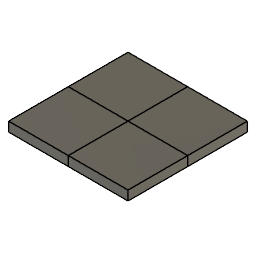
Tile_Base_V1 (Autodesk Fusion 360 design; units mm, degrees)
part number: 2026-04-30-04-34-27-327
Autodesk Fusion 360 part; units mm, degrees
note: some values were not read from the file. Chosen so that the rebuilt part matches the saved one: which bodies a step acts on.
sketch "Sketch1" plane through (0, 0, 0) normal (0, 0, 1) x (1, 0, 0)
  line L0 (-25, 25) -> (25, 25)
  line L1 (25, 25) -> (25, -25)
  line L2 (25, -25) -> (-25, -25)
  line L3 (-25, -25) -> (-25, 25)
  constraint horizontal L0
  constraint vertical L1
  constraint horizontal L2
  constraint vertical L3
extrude "Extrude1" add sketch "Sketch1" along normal blind 5 makes body 1
sketch "Sketch2" plane through (0, -25, 0) normal (0, -1, 0) x (1, 0, 0)
  line L0 (-25, 0) -> (25, 0)
  line L1 (25, 0) -> (25, 5)
  line L2 (25, 5) -> (-25, 5)
  line L3 (-25, 5) -> (-25, 0)
  line L4 (-25, 1) -> (-24, 0)
  line L5 (-24, 0) -> (-25, 0)
  line L6 (-25, 0) -> (-25, 1)
  line L7 (-1, 0) -> (0, 1)
  line L8 (0, 1) -> (1, 0)
  line L9 (1, 0) -> (-1, 0)
  line L10 (24, 0) -> (25, 1)
  line L11 (25, 1) -> (25, 0)
  line L12 (25, 0) -> (24, 0)
  constraint coincident L3 L4.start
  constraint coincident L0 L4.end
  constraint coincident L0.start L3.end
  constraint coincident L0 L7.start
  constraint perpendicular L4 L7
  constraint coincident L0 L8.end
  constraint perpendicular L7 L8
  constraint coincident L0 L10.start
  constraint coincident L1 L10.end
  constraint parallel L7 L10
  constraint coincident L0.end L1.start
extrude "Extrude2" cut sketch "Sketch2" against normal blind 50 contours L0 L3 L4 L5 L6 | L0 L7 L8 L9 | L0 L1 L10 L11 L12 bodies 1
sketch "Sketch3" plane through (25, 0, 0) normal (1, 0, 0) x (0, 1, 0)
  line L0 (-25, 1) -> (25, 1)
  line L1 (25, 1) -> (25, 5)
  line L2 (25, 5) -> (-25, 5)
  line L3 (-25, 5) -> (-25, 1)
  line L4 (-25, 1) -> (-24, 0)
  line L5 (-24, 0) -> (-25, 0)
  line L6 (-25, 0) -> (-25, 1)
  line L7 (-1, 0) -> (0, 1)
  line L8 (0, 1) -> (1, 0)
  line L9 (1, 0) -> (-1, 0)
  line L10 (24, 0) -> (25, 1)
  line L11 (25, 1) -> (25, 0)
  line L12 (24, 0) -> (25, 0)
  constraint coincident L0.start L3.end
  constraint perpendicular L3 L5
  constraint perpendicular L0 L6
  constraint midpoint L0 L7.end
  constraint perpendicular L7 L8
  constraint parallel L0 L9
  constraint coincident L0.end L1.start
  constraint perpendicular L0 L11
  constraint perpendicular L11 L12
extrude "Extrude3" cut sketch "Sketch3" against normal blind 50 contours L10 L11 L12 | L7 L8 L9 | L4 L5 L6 bodies 1
sketch "Sketch4" plane through (25, 0, 0) normal (1, 0, 0) x (0, 1, 0)
  line L0 (-25, 1) -> (0, 1)
  line L1 (0, 1) -> (25, 1)
  line L2 (25, 1) -> (25, 5)
  line L3 (25, 5) -> (-25, 5)
  line L4 (-25, 5) -> (-25, 1)
  line L5 (0, 6) -> (0, 0)
  constraint coincident L5.end origin
  constraint perpendicular L1 L5
split "Split1" by curves path "Sketch4" along L5 bodies 1 makes body 2 at (-8.3333, -8.3333, 5)
sketch "Sketch5" plane through (0, -25, 0) normal (0, -1, 0) x (1, 0, 0)
  line L0 (-25, 1) -> (0, 1)
  line L1 (0, 1) -> (25, 1)
  line L2 (25, 1) -> (25, 5)
  line L3 (25, 5) -> (-25, 5)
  line L4 (-25, 5) -> (-25, 1)
  line L5 (0, 0) -> (0, 6)
  constraint coincident L5.start origin
  constraint perpendicular L3 L5
split "Split2" by curves path "Sketch5" along L5 bodies 2 1 makes body 3 at (8.3333, 8.3333, 5) makes body 4 at (8.3333, -16.6667, 5)
